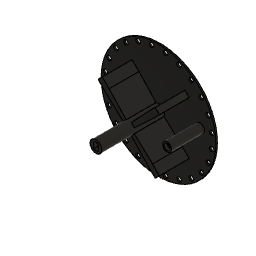
Assembly (Autodesk Fusion 360 archive; units mm, degrees)
design "Hour Wheel 2"
Autodesk Fusion 360 part; units mm, degrees
(part 1 of 2)
sketch "Sketch1" plane through (0, 0, 0) normal (0, 1, 0) x (1, 0, 0)
  circle A0 centre (0, 0) radius 38.5
  circle A1 centre (-4.6989, -35.692) radius 1.5
  circle A2 centre (4.6989, -35.692) radius 1.5
  circle A3 centre (13.7766, -33.2597) radius 1.5
  circle A4 centre (21.9154, -28.5607) radius 1.5
  circle A5 centre (28.5607, -21.9154) radius 1.5
  circle A6 centre (33.2597, -13.7766) radius 1.5
  circle A7 centre (35.692, -4.6989) radius 1.5
  circle A8 centre (35.692, 4.6989) radius 1.5
  circle A9 centre (33.2597, 13.7766) radius 1.5
  circle A10 centre (28.5607, 21.9154) radius 1.5
  circle A11 centre (21.9154, 28.5607) radius 1.5
  circle A12 centre (13.7766, 33.2597) radius 1.5
  circle A13 centre (4.6989, 35.692) radius 1.5
  circle A14 centre (-4.6989, 35.692) radius 1.5
  circle A15 centre (-13.7766, 33.2597) radius 1.5
  circle A16 centre (-21.9154, 28.5607) radius 1.5
  circle A17 centre (-28.5607, 21.9154) radius 1.5
  circle A18 centre (-33.2597, 13.7766) radius 1.5
  circle A19 centre (-35.692, 4.6989) radius 1.5
  circle A20 centre (-35.692, -4.6989) radius 1.5
  circle A21 centre (-33.2597, -13.7766) radius 1.5
  circle A22 centre (-28.5607, -21.9154) radius 1.5
  circle A23 centre (-21.9154, -28.5607) radius 1.5
  circle A24 centre (-13.7766, -33.2597) radius 1.5
  dimension "d1" = 77
  dimension "d2" = 3
  dimension "d3" = 36
  dimension "d5" = 360
  constraint coincident A0.centre origin
  measures "d1" diameter of A0
  measures "d2" diameter of A1
  measures "d3" distance of A0.centre A1.centre
extrude "Extrude1" add sketch "Sketch1" along normal blind 1 makes body 1
sketch "Sketch2" plane through (0, 0, 0) normal (0, 1, 0) x (1, 0, 0)
  line L0 (0, 0) -> (27.6586, 0) construction
  line L1 (0, 0) -> (41.0195, 0) construction
  line L2 (0, 0) -> (31, 0) construction
  line L3 (0, 0) -> (31, 0) construction
  line L4 (-15.9765, 13.148) -> (-13.148, 15.9765)
  line L5 (-14.5622, 14.5622) -> (-15.9765, 13.148)
  line L6 (-14.5622, 14.5622) -> (-13.148, 15.9765)
  line L7 (-15.9765, 13.148) -> (-20.5726, 17.7442)
  line L8 (-20.5726, 17.7442) -> (-17.7442, 20.5726)
  line L9 (-13.148, 15.9765) -> (-17.7442, 20.5726)
  line L10 (-15.9765, -13.148) -> (-20.5726, -17.7442)
  line L11 (-14.5622, -14.5622) -> (-13.148, -15.9765)
  line L12 (-13.148, -15.9765) -> (-17.7442, -20.5726)
  line L13 (-17.7442, -20.5726) -> (-20.5726, -17.7442)
  line L14 (-14.5622, -14.5622) -> (-15.9765, -13.148)
  line L15 (-13.148, -15.9765) -> (-15.9765, -13.148)
  line L16 (13.148, -15.9765) -> (17.7442, -20.5726)
  line L17 (14.5622, -14.5622) -> (15.9765, -13.148)
  line L18 (15.9765, -13.148) -> (20.5726, -17.7442)
  line L19 (20.5726, -17.7442) -> (17.7442, -20.5726)
  line L20 (14.5622, -14.5622) -> (13.148, -15.9765)
  line L21 (15.9765, -13.148) -> (13.148, -15.9765)
  line L22 (15.9765, 13.148) -> (20.5726, 17.7442)
  line L23 (14.5622, 14.5622) -> (13.148, 15.9765)
  line L24 (13.148, 15.9765) -> (17.7442, 20.5726)
  line L25 (17.7442, 20.5726) -> (20.5726, 17.7442)
  line L26 (14.5622, 14.5622) -> (15.9765, 13.148)
  line L27 (13.148, 15.9765) -> (15.9765, 13.148)
  line L28 (-15.9765, 13.148) -> (-3.6903, 1.691)
  line L29 (-15.9765, 13.148) -> (0.824, 13.148) construction
  line L30 (-13.148, 15.9765) -> (-1.7011, 3.7012)
  line L31 (-13.148, 15.9765) -> (3.6363, 15.9765) construction
  line L32 (13.148, 15.9765) -> (1.6437, 3.6396)
  line L33 (13.148, 15.9765) -> (30.0166, 15.9765) construction
  line L34 (15.9765, 13.148) -> (3.7292, 1.7273)
  line L35 (15.9765, 13.148) -> (32.7225, 13.148) construction
  line L36 (-15.9765, -13.148) -> (-3.6901, -1.6909)
  line L37 (-15.9765, -13.148) -> (0.8229, -13.148) construction
  line L38 (-13.148, -15.9765) -> (-1.6943, -3.6938)
  line L39 (-13.148, -15.9765) -> (3.6463, -15.9765) construction
  line L40 (15.9765, -13.148) -> (3.6446, -1.6484)
  line L41 (15.9765, -13.148) -> (32.8382, -13.148) construction
  line L42 (13.148, -15.9765) -> (1.6484, -3.6446)
  line L43 (13.148, -15.9765) -> (30.0097, -15.9765) construction
  arc A0 (3.6463, 1.6445) -> (1.6484, 3.6446) centre (0, 0) ccw
  arc A1 (1.6484, -3.6446) -> (3.6446, -1.6484) centre (0, 0) ccw
  arc A2 (-1.6458, 3.6457) -> (-3.6455, 1.6463) centre (0, 0) ccw
  arc A3 (-3.6455, -1.6463) -> (-1.6461, -3.6456) centre (0, 0) ccw
  line L44 (-3.6455, 1.6463) -> (-3.6903, 1.691)
  line L45 (-3.6901, -1.6909) -> (-3.6455, -1.6463)
  line L46 (1.9993, -0.0019) -> (1.9974, 0)
  line L47 (-1.6458, 3.6457) -> (-1.7011, 3.7012)
  line L48 (3.6463, 1.6445) -> (3.7292, 1.7273)
  line L49 (-1.6943, -3.6938) -> (-1.6461, -3.6456)
  line L50 (1.9993, -0.0019) -> (2.0012, 0)
  dimension "d26" = 2
  dimension "d27" = 2
  dimension "d28" = 6.5
  dimension "d29" = 4
  dimension "d30" = 27.0941
  dimension "d32" = 360
  dimension "d63" = 8
  dimension "d64" = 43
  dimension "d65" = 47
  dimension "d66" = 133
  dimension "d67" = 137
  dimension "d68" = 43
  dimension "d69" = 47
  dimension "d70" = 137
  dimension "d71" = 133
  constraint horizontal L0
  constraint coincident L0.start L1.start
  constraint horizontal L1
  constraint horizontal L2
  constraint horizontal L3
  constraint perpendicular L4 L7
  constraint perpendicular L8 L9
  constraint coincident L4 L5.start
  constraint horizontal L29
  constraint horizontal L31
  constraint horizontal L33
  constraint horizontal L35
  constraint horizontal L37
  constraint horizontal L39
  constraint horizontal L41
  constraint horizontal L43
  constraint coincident L42.end A2
  constraint coincident L32 A0.end
  constraint coincident A2.start L46
  constraint coincident A0.start L49
  constraint concentric A0 A2
  constraint concentric A1 A2
  constraint concentric A2 A3
  constraint collinear L46 L47
  constraint coincident L0 L50.end
  constraint collinear L48 L49
  constraint coincident L0 L46.end
  constraint coincident L46.start L49
  constraint collinear L49 L50
  measures "d26" distance of L5.start L4.start
  measures "d27" distance of L5.start L4.end
  measures "d28" distance of L4.start L7.end
  measures "d29" distance of L7.end L8.end
  measures "d30" distance of L0.start L8
  measures "d63" diameter of A2
  measures "d64" angle of L28 L29
  measures "d65" angle of L30 L31
  measures "d66" angle of L32 L33
  measures "d67" angle of L34 L35
  measures "d68" angle of L36 L37
  measures "d69" angle of L38 L39
  measures "d70" angle of L40 L41
  measures "d71" angle of L42 L43
extrude "Extrude2" add sketch "Sketch2" against normal blind 20 bodies 1
copy_body "Body->Comp1" bodies 1 removing the originals makes body 2 in component "Wheel"
sketch "Sketch3" plane through (0, 0, 0) normal (0, 1, 0) x (1, 0, 0)
  circle A0 centre (0, 0) radius 4
  dimension "d37" = 8
  constraint coincident A0.centre origin
  measures "d37" diameter of A0
extrude "Extrude1'" add sketch "Sketch3" against normal blind 42 bodies 2 in component "Wheel"
sketch "Sketch4" plane through (0, 0, 0) normal (0, 1, 0) x (1, 0, 0)
  line L0 (1.5, -2) -> (1.5, 2)
  line L1 (-1.5, 2) -> (-1.5, -2)
  arc A0 (-1.5, -2) -> (1.5, -2) centre (0, 0) ccw
  arc A1 (1.5, 2) -> (-1.5, 2) centre (0, 0) ccw
  dimension "d40" = 5
  dimension "d41" = 3
  dimension "d42" = 4
  constraint coincident A0.centre A1.centre
  constraint vertical L0
  constraint vertical L1
  constraint concentric A0 A1
  measures "d40" diameter of A0
  measures "d41" distance of L1.end L0.start
  measures "d42" distance of L1.end L1.start
extrude "Extrude2'" cut sketch "Sketch4" along normal blind 6.5 from surface at -42 bodies 2 in component "Wheel"
sketch "Sketch8" plane through (0, 0, 0) normal (0, 1, 0) x (1, 0, 0)
  line L0 (1.5, -1.5) -> (-1.5, -1.5)
  line L1 (-1.5, -1.5) -> (-1.5, 1.5)
  line L2 (-1.5, 1.5) -> (1.5, 1.5)
  line L3 (1.5, 1.5) -> (1.5, -1.5)
  dimension "d87" = 3
  dimension "d88" = 3
  dimension "d89" = 1.5
  dimension "d90" = 1.5
  constraint horizontal L0
  constraint vertical L1
  constraint horizontal L2
  constraint vertical L3
  measures "d87" distance of L0.start L0.end
  measures "d88" distance of L0.start L2.end
  measures "d89" distance of origin L3
  measures "d90" distance of origin L0
sketch "Sketch9" plane through (0, 0, 0) normal (0, 1, 0) x (1, 0, 0)
  circle A0 centre (0, 0) radius 10
  line L0 (0.6946, -3.9392) -> (1.5628, -8.8633)
  line L1 (4, 0) -> (9, 0) construction
  line L2 (3.9392, -0.6946) -> (8.8633, -1.5628)
  line L3 (4, 0) -> (9, 0) construction
  line L4 (-0.6946, -3.9392) -> (-1.5628, -8.8633)
  line L5 (4, 0) -> (9, 0) construction
  line L6 (-3.9392, -0.6946) -> (-8.8633, -1.5628)
  line L7 (4, 0) -> (9, 0) construction
  line L8 (-3.9392, 0.6946) -> (-8.8633, 1.5628)
  line L9 (4, 0) -> (9, 0) construction
  line L10 (3.9392, 0.6946) -> (8.8633, 1.5628)
  line L11 (4, 0) -> (9, 0) construction
  line L12 (-0.6946, 3.9392) -> (-1.5628, 8.8633)
  line L13 (0.6946, 3.9392) -> (1.5628, 8.8633)
  arc A1 (8.8633, 1.5628) -> (1.5628, 8.8633) centre (0, 0) ccw
  arc A2 (-1.5628, 8.8633) -> (-8.8633, 1.5628) centre (0, 0) ccw
  arc A3 (-8.8633, -1.5628) -> (-1.5628, -8.8633) centre (0, 0) ccw
  arc A4 (1.5628, -8.8633) -> (8.8633, -1.5628) centre (0, 0) ccw
  arc A5 (3.9392, 0.6946) -> (0.6946, 3.9392) centre (0, 0) ccw
  arc A6 (-0.6946, 3.9392) -> (-3.9392, 0.6946) centre (0, 0) ccw
  arc A7 (-3.9392, -0.6946) -> (-0.6946, -3.9392) centre (0, 0) ccw
  arc A8 (0.6946, -3.9392) -> (3.9392, -0.6946) centre (0, 0) ccw
  dimension "d81" = 80
  dimension "d82" = 10
  dimension "d83" = 100
  dimension "d84" = 170
  dimension "d85" = 170
  dimension "d86" = 10
  constraint horizontal L1
  constraint horizontal L3
  constraint horizontal L5
  constraint horizontal L7
  constraint horizontal L9
  constraint horizontal L11
  constraint coincident L12.end A1
  constraint parallel L0 L12
  constraint perpendicular L8 L13
  constraint concentric A1 A2
  constraint concentric A2 A3
  constraint concentric A3 A4
  constraint concentric A1 A5
  constraint coincident L4.start A5
  constraint coincident L6.start A5
  constraint coincident L8.start A5
  constraint coincident L12.start A5
  constraint concentric A5 A6
  constraint concentric A6 A7
  constraint coincident A0.centre A1.centre
  measures "d81" angle of L0 L1
  measures "d82" angle of L2 L3
  measures "d83" angle of L4 L5
  measures "d84" angle of L6 L7
  measures "d85" angle of L8 L9
  measures "d86" angle of L10 L11
extrude "Extrude5" cut sketch "Sketch8" against normal blind 10 from surface at 2 bodies 2 in component "Wheel"
sketch "Sketch10" plane through (0, 0, 0) normal (0, -1, 0) x (1, 0, 0)
  arc A0 (-1.6458, -3.6457) -> (1.6484, -3.6446) centre (0, 0) ccw
  line L0 (-1.6458, -3.6457) -> (-1.7011, -3.7012)
  line L1 (-1.7011, -3.7012) -> (-13.148, -15.9765)
  line L2 (-13.148, -15.9765) -> (-17.7442, -20.5726)
  line L3 (-17.7442, -20.5726) -> (-20.5726, -17.7442)
  line L4 (-20.5726, -17.7442) -> (-15.9765, -13.148)
  line L5 (-15.9765, -13.148) -> (-3.6903, -1.691)
  line L6 (-3.6903, -1.691) -> (-3.6455, -1.6463)
  arc A1 (-3.6455, 1.6463) -> (-3.6455, -1.6463) centre (0, 0) ccw
  line L7 (-3.6455, 1.6463) -> (-3.6901, 1.6909)
  line L8 (-3.6901, 1.6909) -> (-15.9765, 13.148)
  line L9 (-15.9765, 13.148) -> (-20.5726, 17.7442)
  line L10 (-20.5726, 17.7442) -> (-17.7442, 20.5726)
  line L11 (-17.7442, 20.5726) -> (-13.148, 15.9765)
  line L12 (-13.148, 15.9765) -> (-1.6943, 3.6938)
  line L13 (-1.6943, 3.6938) -> (-1.6461, 3.6456)
  arc A2 (1.6484, 3.6446) -> (-1.6461, 3.6456) centre (0, 0) ccw
  line L14 (1.6484, 3.6446) -> (13.148, 15.9765)
  line L15 (13.148, 15.9765) -> (17.7442, 20.5726)
  line L16 (17.7442, 20.5726) -> (20.5726, 17.7442)
  line L17 (20.5726, 17.7442) -> (15.9765, 13.148)
  line L18 (15.9765, 13.148) -> (3.6446, 1.6484)
  arc A3 (3.6463, -1.6445) -> (3.6446, 1.6484) centre (0, 0) ccw
  line L19 (3.6463, -1.6445) -> (3.7292, -1.7273)
  line L20 (3.7292, -1.7273) -> (15.9765, -13.148)
  line L21 (15.9765, -13.148) -> (20.5726, -17.7442)
  line L22 (20.5726, -17.7442) -> (17.7442, -20.5726)
  line L23 (17.7442, -20.5726) -> (13.148, -15.9765)
  line L24 (13.148, -15.9765) -> (1.6484, -3.6446)
  circle A4 centre (-35.692, -4.6989) radius 1.5
  circle A5 centre (-33.2597, 13.7766) radius 1.5
  circle A6 centre (-28.5607, 21.9154) radius 1.5
  circle A7 centre (-21.9154, 28.5607) radius 1.5
  circle A8 centre (-13.7766, 33.2597) radius 1.5
  circle A9 centre (-35.692, 4.6989) radius 1.5
  circle A10 centre (-33.2597, -13.7766) radius 1.5
  circle A11 centre (-28.5607, -21.9154) radius 1.5
  circle A12 centre (-21.9154, -28.5607) radius 1.5
  circle A13 centre (-13.7766, -33.2597) radius 1.5
  circle A14 centre (4.6989, -35.692) radius 1.5
  circle A15 centre (-4.6989, -35.692) radius 1.5
  circle A16 centre (13.7766, -33.2597) radius 1.5
  circle A17 centre (21.9154, -28.5607) radius 1.5
  circle A18 centre (28.5607, -21.9154) radius 1.5
  circle A19 centre (33.2597, -13.7766) radius 1.5
  circle A20 centre (35.692, -4.6989) radius 1.5
  circle A21 centre (35.692, 4.6989) radius 1.5
  circle A22 centre (33.2597, 13.7766) radius 1.5
  circle A23 centre (28.5607, 21.9154) radius 1.5
  circle A24 centre (21.9154, 28.5607) radius 1.5
  circle A25 centre (13.7766, 33.2597) radius 1.5
  circle A26 centre (4.6989, 35.692) radius 1.5
  circle A27 centre (-4.6989, 35.692) radius 1.5
  circle A28 centre (0, 0) radius 38.5
  circle A29 centre (27.7605, 3.6547) radius 3
  dimension "d91" = 8
  dimension "d92" = 6
  measures "d91" distance of A21.centre A29.centre
  measures "d92" diameter of A29
extrude "Extrude7" add sketch "Sketch10" along normal blind 22 contours A29 bodies 2 in component "Wheel"
sketch "Sketch11" plane through (0, -22, 0) normal (0, -1, 0) x (1, 0, 0)
  circle A0 centre (27.7605, 3.6547) radius 3
  circle A1 centre (27.7605, 3.6547) radius 2
  dimension "d96" = 4
  constraint concentric A0 A1
  measures "d96" diameter of A1
extrude "Extrude8" cut sketch "Sketch11" against normal blind 2 contours A1 bodies 2 in component "Wheel"
component "Wheel" placed x (1, 0, 0) y (0, 1, 0) z (0, 0, 1) at (0, 0, 0)

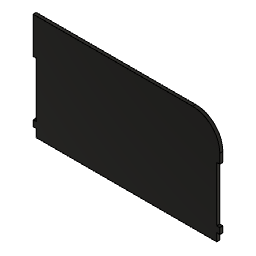
design "Minute Flap"
Autodesk Fusion 360 part; units mm, degrees
sketch "Sketch1" plane through (0, 0, 0) normal (0, 1, 0) x (1, 0, 0)
  line L0 (1, 0) -> (61, 0)
  line L1 (53, -35) -> (0, -35)
  arc A0 (53, -35) -> (62, -26) centre (53, -26) ccw
  line L2 (0, -2.6) -> (1, -2.6)
  line L3 (1, -4.6) -> (0, -4.6)
  line L4 (0, -4.6) -> (0, -2.6)
  line L5 (1, -2.6) -> (1, 0)
  line L6 (1, -4.6) -> (1, -22.85)
  line L7 (1, -22.85) -> (0, -22.85)
  line L8 (0, -35) -> (0, -22.85)
  line L9 (0, -4.6) -> (0, -2.6)
  line L10 (61, -22.85) -> (62, -22.85)
  line L11 (61, -4.6) -> (62, -4.6)
  line L12 (61, -2.6) -> (62, -2.6)
  line L13 (61, -2.6) -> (61, 0)
  line L14 (61, -4.6) -> (61, -22.85)
  line L15 (62, -2.6) -> (62, -4.6)
  line L16 (62, -22.85) -> (62, -26)
  dimension "d2" = 35
  dimension "d3" = 9
  dimension "d4" = 1
  dimension "d5" = 2
  dimension "d6" = 2.6
  dimension "d7" = 18.25
  dimension "d9" = 2.6
  dimension "d10" = 2
  dimension "d11" = 18.25
  dimension "d14" = 53
  dimension "d15" = 1
  dimension "d16" = 1
  constraint horizontal L0
  constraint vertical L15
  constraint horizontal L1
  constraint vertical L8
  constraint tangent L1 A0
  constraint tangent A0 L15
  constraint horizontal L2
  constraint horizontal L3
  constraint vertical L4
  constraint perpendicular L0 L5
  constraint perpendicular L3 L6
  constraint perpendicular L7 L8
  constraint collinear L8 L9
  constraint coincident L10.end L15
  constraint perpendicular L10 L15
  constraint perpendicular L11 L15
  constraint perpendicular L12 L15
  constraint perpendicular L0 L13
  constraint perpendicular L10 L14
  constraint collinear L15 L16
  measures "d2" distance of origin L1.end
  measures "d3" radius of A0
  measures "d4" distance of L2.start L2.end
  measures "d5" distance of L2.start L3.end
  measures "d6" distance of L0 L2
  measures "d7" distance of L3.start L6.end
  measures "d9" distance of L12.start L0.end
  measures "d10" distance of L12.start L11.start
  measures "d11" distance of L11.start L10.start
  measures "d14" distance of L1.end L1.start
  measures "d15" distance of L10.end L10.start
  measures "d16" distance of L12.end L12.start
extrude "Extrude1" add sketch "Sketch1" along normal blind 1 makes body 1
copy_body "Body->Comp1" bodies 1 removing the originals makes body 2 in component "Flap"
component "Flap" placed x (1, 0, 0) y (0, 1, 0) z (0, 0, 1) at (0, 0, 0)

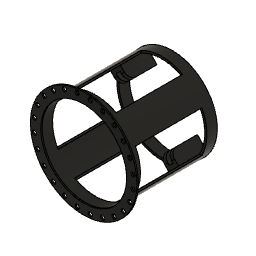
design "Hour Wheel 1"
Autodesk Fusion 360 part; units mm, degrees
sketch "Sketch1" plane through (0, 0, 0) normal (0, 1, 0) x (1, 0, 0)
  circle A0 centre (49.9693, -49.8433) radius 38.5
  circle A1 centre (45.2704, -85.5353) radius 1.5
  circle A2 centre (54.6683, -85.5353) radius 1.5
  circle A3 centre (63.7459, -83.103) radius 1.5
  circle A4 centre (71.8847, -78.404) radius 1.5
  circle A5 centre (78.53, -71.7587) radius 1.5
  circle A6 centre (83.229, -63.6199) radius 1.5
  circle A7 centre (85.6613, -54.5423) radius 1.5
  circle A8 centre (85.6613, -45.1444) radius 1.5
  circle A9 centre (83.229, -36.0667) radius 1.5
  circle A10 centre (78.53, -27.9279) radius 1.5
  circle A11 centre (71.8847, -21.2826) radius 1.5
  circle A12 centre (63.7459, -16.5837) radius 1.5
  circle A13 centre (54.6683, -14.1513) radius 1.5
  circle A14 centre (45.2704, -14.1513) radius 1.5
  circle A15 centre (36.1927, -16.5837) radius 1.5
  circle A16 centre (28.0539, -21.2826) radius 1.5
  circle A17 centre (21.4086, -27.9279) radius 1.5
  circle A18 centre (16.7096, -36.0667) radius 1.5
  circle A19 centre (14.2773, -45.1444) radius 1.5
  circle A20 centre (14.2773, -54.5423) radius 1.5
  circle A21 centre (16.7096, -63.6199) radius 1.5
  circle A22 centre (21.4086, -71.7587) radius 1.5
  circle A23 centre (28.0539, -78.404) radius 1.5
  circle A24 centre (36.1927, -83.103) radius 1.5
  circle A25 centre (49.9693, -49.8433) radius 31
  dimension "d1" = 77
  dimension "d2" = 3
  dimension "d3" = 36
  dimension "d5" = 360
  dimension "d6" = 62
  constraint concentric A0 A25
  measures "d1" diameter of A0
  measures "d2" diameter of A1
  measures "d3" distance of A0.centre A1.centre
  measures "d6" diameter of A25
extrude "Extrude1" add sketch "Sketch1" along normal blind 1 makes body 1
sketch "Sketch2" plane through (0, 0, 0) normal (0, -1, 0) x (1, 0, 0)
  circle A0 centre (16.7096, 63.6199) radius 1.5
  circle A1 centre (21.4086, 71.7587) radius 1.5
  circle A2 centre (28.0539, 78.404) radius 1.5
  circle A3 centre (36.1927, 83.103) radius 1.5
  circle A4 centre (49.9693, 49.8433) radius 31
  circle A5 centre (54.6683, 14.1513) radius 1.5
  circle A6 centre (45.2704, 14.1513) radius 1.5
  circle A7 centre (36.1927, 16.5837) radius 1.5
  circle A8 centre (28.0539, 21.2826) radius 1.5
  circle A9 centre (21.4086, 27.9279) radius 1.5
  circle A10 centre (16.7096, 36.0667) radius 1.5
  circle A11 centre (14.2773, 45.1444) radius 1.5
  circle A12 centre (14.2773, 54.5423) radius 1.5
  circle A13 centre (63.7459, 16.5837) radius 1.5
  circle A14 centre (71.8847, 21.2826) radius 1.5
  circle A15 centre (78.53, 27.9279) radius 1.5
  circle A16 centre (83.229, 36.0667) radius 1.5
  circle A17 centre (85.6613, 45.1444) radius 1.5
  circle A18 centre (85.6613, 54.5423) radius 1.5
  circle A19 centre (83.229, 63.6199) radius 1.5
  circle A20 centre (78.53, 71.7587) radius 1.5
  circle A21 centre (71.8847, 78.404) radius 1.5
  circle A22 centre (63.7459, 83.103) radius 1.5
  circle A23 centre (54.6683, 85.5353) radius 1.5
  circle A24 centre (45.2704, 85.5353) radius 1.5
  circle A25 centre (49.9693, 49.8433) radius 38.5
sketch "Sketch3" plane through (0, 0, 0) normal (0, -1, 0) x (1, 0, 0)
  circle A0 centre (50, 50) radius 32.5
  circle A1 centre (50, 50) radius 31
  dimension "d10" = 65
  dimension "d22" = 62
  constraint concentric A0 A1
  measures "d10" diameter of A0
  measures "d22" diameter of A1
extrude "Extrude4" add sketch "Sketch3" against normal blind 63 from surface at -1 separate body makes body 2
sketch "Sketch5" plane through (0, 0, 0) normal (1, 0, 0) x (0, 1, 0)
  line L0 (8.5, 64.8433) -> (56.5, 64.8433)
  line L1 (56.5, 64.8433) -> (56.5, 34.8433)
  line L2 (56.5, 34.8433) -> (8.5, 34.8433)
  line L3 (8.5, 34.8433) -> (8.5, 64.8433)
  line L4 (1, 11.5) -> (1, 50)
  line L5 (1, 11.3433) -> (1, 88.3433)
  point P0 (1, 49.8433)
  dimension "d23" = 48
  dimension "d24" = 30
  dimension "d25" = 38.5
  dimension "d26" = 15
  dimension "d29" = 7.5
  constraint horizontal L0
  constraint vertical L1
  constraint horizontal L2
  constraint vertical L3
  constraint vertical L4
  measures "d23" distance of L0.start L0.end
  measures "d24" distance of L0.end L1.end
  measures "d25" distance of L4.start L4.end
  measures "d26" vertical distance of L2.end P0
  measures "d29" distance of L3 L5
extrude "Extrude5" cut sketch "Sketch5" along normal blind 100 bodies 2
sketch "Sketch6" plane through (0, 0, 0) normal (0, 0, 1) x (1, 0, 0)
  line L0 (34.9693, 56.5) -> (64.9693, 56.5)
  line L1 (64.9693, 56.5) -> (64.9693, 8.5)
  line L2 (64.9693, 8.5) -> (34.9693, 8.5)
  line L3 (34.9693, 8.5) -> (34.9693, 56.5)
  line L4 (88.4693, 1) -> (11.4693, 1)
  line L5 (88.4693, 1) -> (49.9693, 1)
  dimension "d30" = 30
  dimension "d31" = 48
  dimension "d32" = 7.5
  dimension "d33" = 38.5
  dimension "d34" = 15
  constraint horizontal L0
  constraint vertical L1
  constraint horizontal L2
  constraint vertical L3
  constraint coincident L4.start L5.start
  constraint parallel L4 L5
  measures "d30" distance of L0.start L0.end
  measures "d31" distance of L0.end L1.end
  measures "d32" distance of L2 L4
  measures "d33" distance of L4.start L5.end
  measures "d34" horizontal distance of L1.end L5.end
extrude "Extrude6" cut sketch "Sketch6" along normal blind 95 bodies 2
copy_body "Body->Comp5" bodies 1 removing the originals makes body 3 in component "Wheel"
copy_body "Body->Comp6" bodies 2 removing the originals makes body 4 in component "Axis"
sketch "Sketch11" plane through (0, 64, 0) normal (0, 1, 0) x (-1, 0, 0)
  circle A0 centre (0.0307, -0.1567) radius 31
  circle A1 centre (0.0307, -0.1567) radius 32.5
  line L0 (0.0307, -0.1567) -> (31.0307, -0.1567) construction
  line L1 (18.1285, -25.3255) -> (11.0574, -18.2544)
  line L2 (25.1995, -18.2544) -> (18.1285, -11.1834)
  arc A2 (18.1285, -25.3255) -> (25.1995, -18.2544) centre (0.0307, -0.1567) ccw
  line L3 (25.1995, -18.2544) -> (18.1285, -11.1834)
  line L4 (13.1787, -16.1331) -> (17.7749, -20.7293)
  line L5 (17.7749, -20.7293) -> (20.6033, -17.9009)
  line L6 (20.6033, -17.9009) -> (16.0071, -13.3047)
  line L7 (18.1285, -11.1834) -> (16.0071, -13.3047)
  line L8 (13.1787, -16.1331) -> (11.0574, -18.2544)
  line L9 (18.1285, 25.0122) -> (11.0574, 17.9411)
  line L10 (16.0071, 12.9914) -> (18.1285, 10.87)
  line L11 (17.7749, 20.416) -> (13.1787, 15.8198)
  arc A3 (25.1995, 17.9411) -> (18.1285, 25.0122) centre (0.0307, -0.1567) ccw
  line L12 (20.6033, 17.5875) -> (17.7749, 20.416)
  line L13 (11.0574, 17.9411) -> (13.1787, 15.8198)
  line L14 (25.1995, 17.9411) -> (18.1285, 10.87)
  line L15 (16.0071, 12.9914) -> (20.6033, 17.5875)
  line L16 (18.1285, 25.0122) -> (11.0574, 17.9411)
  line L17 (-25.1381, 17.9411) -> (-18.0671, 10.87)
  line L18 (-13.1173, 15.8198) -> (-10.996, 17.9411)
  line L19 (-20.542, 17.5875) -> (-15.9458, 12.9914)
  arc A4 (-18.0671, 25.0122) -> (-25.1381, 17.9411) centre (0.0307, -0.1567) ccw
  line L20 (-17.7135, 20.416) -> (-20.542, 17.5875)
  line L21 (-18.0671, 10.87) -> (-15.9458, 12.9914)
  line L22 (-18.0671, 25.0122) -> (-10.996, 17.9411)
  line L23 (-13.1173, 15.8198) -> (-17.7135, 20.416)
  line L24 (-25.1381, 17.9411) -> (-18.0671, 10.87)
  line L25 (-18.0671, -25.3255) -> (-10.996, -18.2544)
  line L26 (-15.9458, -13.3047) -> (-18.0671, -11.1834)
  line L27 (-17.7135, -20.7293) -> (-13.1173, -16.1331)
  arc A5 (-25.1381, -18.2544) -> (-18.0671, -25.3255) centre (0.0307, -0.1567) ccw
  line L28 (-20.542, -17.9009) -> (-17.7135, -20.7293)
  line L29 (-10.996, -18.2544) -> (-13.1173, -16.1331)
  line L30 (-25.1381, -18.2544) -> (-18.0671, -11.1834)
  line L31 (-15.9458, -13.3047) -> (-20.542, -17.9009)
  line L32 (-18.0671, -25.3255) -> (-10.996, -18.2544)
  dimension "d107" = 10
  dimension "d108" = 6.5
  dimension "d109" = 4
  dimension "d110" = 3
  dimension "d111" = 3
  dimension "d112" = 6.5
  dimension "d114" = 360
  constraint concentric A0 A2
  constraint horizontal L0
  constraint coincident A0.centre A1.centre
  constraint coincident A0 L2.start
  constraint coincident A0 L1.start
  constraint parallel L2 L3
  constraint perpendicular L1 L7
  constraint coincident L4.start L7
  constraint perpendicular L4 L7
  constraint perpendicular L6 L7
  constraint collinear L7 L8
  measures "d107" distance of L2.start L2.end
  measures "d108" distance of L4.start L4.end
  measures "d109" distance of L4.end L5.end
  measures "d110" distance of L1 L4
  measures "d111" distance of L2 L6
  measures "d112" distance of L5.end L6.end
extrude "Extrude1'" add sketch "Sketch11" against normal blind 20 contours A0 L9 L10 L11 A3 L12 L13 L14 L15 L16 | A0 L1 L2 A2 L3 L4 L5 L6 L7 L8 | A0 L17 L18 L19 A4 L20 L21 L22 L23 L24 | A0 L25 L26 L27 A5 L28 L29 L30 L31 L32 sketch seen with x (1, 0, 0) y (0, 1, 0) z (0, 0, 1) at (50.0307, 0, 50.1567) bodies 4 in component "Axis"
fillet "Fillet1" radius 5 8 edges at (37.9126, 44, 67.0371) (32.9629, 44, 62.0874) (32.9629, 44, 37.9126) (37.9126, 44, 32.9629) (67.0371, 44, 37.9126) (62.0874, 44, 32.9629) (62.0874, 44, 67.0371) (67.0371, 44, 62.0874) on bodies 4 in component "Axis"
component "Wheel" placed x (1, 0, 0) y (0, 1, 0) z (0, 0, 1) at (-50, 0, -50)
component "Axis" placed x (1, 0, 0) y (0, 1, 0) z (0, 0, 1) at (-50.0307, 0, -50.1567)
equation "d25 = ( 77 / 2 ) * 1 mm"
equation "d33 = ( 77 / 2 ) * 1 mm"

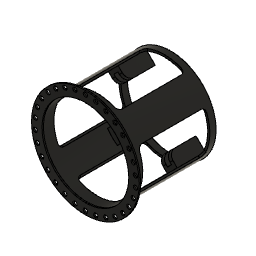
design "Minute Wheel 1"
Autodesk Fusion 360 part; units mm, degrees
sketch "Sketch1" plane through (0, 0, 0) normal (0, 1, 0) x (1, 0, 0)
  circle A0 centre (50, -49.5) radius 38.5
  circle A1 centre (50, -49.5) radius 31
  circle A2 centre (50, -85.5) radius 1.5
  circle A3 centre (57.4848, -84.7133) radius 1.5
  circle A4 centre (64.6425, -82.3876) radius 1.5
  circle A5 centre (71.1603, -78.6246) radius 1.5
  circle A6 centre (76.7532, -73.5887) radius 1.5
  circle A7 centre (81.1769, -67.5) radius 1.5
  circle A8 centre (84.238, -60.6246) radius 1.5
  circle A9 centre (85.8028, -53.263) radius 1.5
  circle A10 centre (85.8028, -45.737) radius 1.5
  circle A11 centre (84.238, -38.3754) radius 1.5
  circle A12 centre (81.1769, -31.5) radius 1.5
  circle A13 centre (76.7532, -25.4113) radius 1.5
  circle A14 centre (71.1603, -20.3754) radius 1.5
  circle A15 centre (64.6425, -16.6124) radius 1.5
  circle A16 centre (57.4848, -14.2867) radius 1.5
  circle A17 centre (50, -13.5) radius 1.5
  circle A18 centre (42.5152, -14.2867) radius 1.5
  circle A19 centre (35.3575, -16.6124) radius 1.5
  circle A20 centre (28.8397, -20.3754) radius 1.5
  circle A21 centre (23.2468, -25.4113) radius 1.5
  circle A22 centre (18.8231, -31.5) radius 1.5
  circle A23 centre (15.762, -38.3754) radius 1.5
  circle A24 centre (14.1972, -45.737) radius 1.5
  circle A25 centre (14.1972, -53.263) radius 1.5
  circle A26 centre (15.762, -60.6246) radius 1.5
  circle A27 centre (18.8231, -67.5) radius 1.5
  circle A28 centre (23.2468, -73.5887) radius 1.5
  circle A29 centre (28.8397, -78.6246) radius 1.5
  circle A30 centre (35.3575, -82.3876) radius 1.5
  circle A31 centre (42.5152, -84.7133) radius 1.5
  dimension "d1" = 77
  dimension "d6" = 62
  dimension "d86" = 3
  dimension "d87" = 36
  dimension "d89" = 360
  constraint concentric A0 A1
  measures "d1" diameter of A0
  measures "d6" diameter of A1
  measures "d86" diameter of A2
  measures "d87" distance of A0.centre A2.centre
extrude "Extrude1" add sketch "Sketch1" along normal blind 1 makes body 1
sketch "Sketch2" plane through (0, 0, 0) normal (0, -1, 0) x (1, 0, 0)
  circle A0 centre (50, 49.5) radius 31
  circle A1 centre (50, 49.5) radius 38.5
  circle A2 centre (18.8231, 67.5) radius 1.5
  circle A3 centre (35.3575, 82.3876) radius 1.5
  circle A4 centre (64.6425, 16.6124) radius 1.5
  circle A5 centre (23.2468, 73.5887) radius 1.5
  circle A6 centre (28.8397, 78.6246) radius 1.5
  circle A7 centre (14.1972, 53.263) radius 1.5
  circle A8 centre (15.762, 60.6246) radius 1.5
  circle A9 centre (42.5152, 14.2867) radius 1.5
  circle A10 centre (50, 13.5) radius 1.5
  circle A11 centre (57.4848, 14.2867) radius 1.5
  circle A12 centre (42.5152, 84.7133) radius 1.5
  circle A13 centre (35.3575, 16.6124) radius 1.5
  circle A14 centre (28.8397, 20.3754) radius 1.5
  circle A15 centre (23.2468, 25.4113) radius 1.5
  circle A16 centre (18.8231, 31.5) radius 1.5
  circle A17 centre (15.762, 38.3754) radius 1.5
  circle A18 centre (14.1972, 45.737) radius 1.5
  circle A19 centre (71.1603, 20.3754) radius 1.5
  circle A20 centre (76.7532, 25.4113) radius 1.5
  circle A21 centre (81.1769, 31.5) radius 1.5
  circle A22 centre (84.238, 38.3754) radius 1.5
  circle A23 centre (85.8028, 45.737) radius 1.5
  circle A24 centre (85.8028, 53.263) radius 1.5
  circle A25 centre (84.238, 60.6246) radius 1.5
  circle A26 centre (81.1769, 67.5) radius 1.5
  circle A27 centre (76.7532, 73.5887) radius 1.5
  circle A28 centre (71.1603, 78.6246) radius 1.5
  circle A29 centre (64.6425, 82.3876) radius 1.5
  circle A30 centre (57.4848, 84.7133) radius 1.5
  circle A31 centre (50, 85.5) radius 1.5
sketch "Sketch3" plane through (0, 0, 0) normal (0, -1, 0) x (1, 0, 0)
  circle A0 centre (50, 50) radius 32.5
  circle A1 centre (50, 50) radius 31
  dimension "d10" = 65
  dimension "d22" = 62
  constraint concentric A0 A1
  measures "d10" diameter of A0
  measures "d22" diameter of A1
extrude "Extrude4" add sketch "Sketch3" against normal blind 60 from surface at -1 separate body makes body 2
sketch "Sketch5" plane through (0, 0, 0) normal (1, 0, 0) x (0, 1, 0)
  line L0 (11.5, 64.5) -> (53.5, 64.5)
  line L1 (56.5, 61.5) -> (56.5, 37.5)
  line L2 (53.5, 34.5) -> (11.5, 34.5)
  line L3 (8.5, 37.5) -> (8.5, 61.5)
  line L4 (1, 11.5) -> (1, 50)
  line L5 (1, 11) -> (1, 88)
  arc A0 (56.5, 61.5) -> (53.5, 64.5) centre (53.5, 61.5) ccw
  arc A1 (11.5, 64.5) -> (8.5, 61.5) centre (11.5, 61.5) ccw
  arc A2 (53.5, 34.5) -> (56.5, 37.5) centre (53.5, 37.5) ccw
  arc A3 (8.5, 37.5) -> (11.5, 34.5) centre (11.5, 37.5) ccw
  point P0 (8.5, 64.5)
  point P1 (56.5, 64.5)
  point P2 (56.5, 34.5)
  point P3 (8.5, 34.5)
  point P4 (1, 49.5)
  dimension "d23" = 48
  dimension "d24" = 30
  dimension "d25" = 38.5
  dimension "d26" = 15
  dimension "d29" = 7.5
  dimension "d94" = 3
  dimension "d95" = 3
  dimension "d96" = 3
  dimension "d97" = 3
  constraint horizontal L0
  constraint vertical L1
  constraint horizontal L2
  constraint vertical L3
  constraint vertical L4
  constraint coincident P1 L0
  constraint coincident P1 L1
  constraint tangent L0 A0
  constraint tangent L1 A0
  constraint coincident P0 L0
  constraint coincident P0 L3
  constraint tangent L0 A1
  constraint tangent L3 A1
  constraint coincident P2 L1
  constraint coincident P2 L2
  constraint tangent L1 A2
  constraint tangent L2 A2
  constraint coincident P3 L3
  constraint coincident P3 L2
  constraint tangent L3 A3
  constraint tangent L2 A3
  measures "d23" distance of P0 P1
  measures "d24" distance of P1 P2
  measures "d25" distance of L4.start L4.end
  measures "d26" vertical distance of P3 P4
  measures "d29" distance of L3 L5
  measures "d94" radius of A0
  measures "d95" radius of A1
  measures "d96" radius of A2
  measures "d97" radius of A3
extrude "Extrude5" cut sketch "Sketch5" along normal blind 100 bodies 2
sketch "Sketch6" plane through (0, 0, 0) normal (0, 0, 1) x (1, 0, 0)
  line L0 (38, 56.5) -> (62, 56.5)
  line L1 (65, 53.5) -> (65, 11.5)
  line L2 (62, 8.5) -> (38, 8.5)
  line L3 (35, 11.5) -> (35, 53.5)
  line L4 (88.5, 1) -> (11.5, 1)
  line L5 (88.5, 1) -> (50, 1)
  arc A0 (35, 11.5) -> (38, 8.5) centre (38, 11.5) ccw
  arc A1 (62, 8.5) -> (65, 11.5) centre (62, 11.5) ccw
  arc A2 (38, 56.5) -> (35, 53.5) centre (38, 53.5) ccw
  arc A3 (65, 53.5) -> (62, 56.5) centre (62, 53.5) ccw
  point P0 (35, 56.5)
  point P1 (65, 56.5)
  point P2 (65, 8.5)
  dimension "d30" = 30
  dimension "d31" = 48
  dimension "d32" = 7.5
  dimension "d33" = 38.5
  dimension "d34" = 15
  dimension "d90" = 3
  dimension "d91" = 3
  dimension "d92" = 3
  dimension "d93" = 3
  constraint horizontal L0
  constraint vertical L1
  constraint horizontal L2
  constraint vertical L3
  constraint coincident L4.start L5.start
  constraint parallel L4 L5
  constraint tangent L3 A0
  constraint tangent L2 A0
  constraint coincident P2 L1
  constraint coincident P2 L2
  constraint tangent L1 A1
  constraint tangent L2 A1
  constraint coincident P0 L0
  constraint coincident P0 L3
  constraint tangent L0 A2
  constraint tangent L3 A2
  constraint coincident P1 L0
  constraint coincident P1 L1
  constraint tangent L0 A3
  constraint tangent L1 A3
  measures "d30" distance of P0 P1
  measures "d31" distance of P1 P2
  measures "d32" distance of L2 L4
  measures "d33" distance of L4.start L5.end
  measures "d34" horizontal distance of P2 L5.end
  measures "d90" radius of A0
  measures "d91" radius of A1
  measures "d92" radius of A2
  measures "d93" radius of A3
extrude "Extrude6" cut sketch "Sketch6" along normal blind 95 bodies 2
copy_body "Body->Comp5" bodies 2 removing the originals makes body 3 in component "Axis"
copy_body "Body->Comp6" bodies 1 removing the originals makes body 4 in component "Wheel"
sketch "Sketch9" plane through (0, 0, 0) normal (0, 1, 0) x (1, 0, 0)
  line L0 (50, -50) -> (81, -50) construction
  line L1 (31.9022, -24.8312) -> (38.9733, -31.9022)
  line L2 (24.8312, -31.9022) -> (31.9022, -38.9733)
  line L3 (36.852, -34.0235) -> (32.2558, -29.4274)
  line L4 (32.2558, -29.4274) -> (29.4274, -32.2558)
  line L5 (29.4274, -32.2558) -> (34.0235, -36.852)
  line L6 (31.9022, -38.9733) -> (34.0235, -36.852)
  line L7 (36.852, -34.0235) -> (38.9733, -31.9022)
  arc A0 (31.9022, -24.8312) -> (24.8312, -31.9022) centre (50, -50) ccw
  line L8 (31.9022, -75.1688) -> (38.9733, -68.0978)
  line L9 (32.2558, -70.5726) -> (36.852, -65.9765)
  line L10 (29.4274, -67.7442) -> (32.2558, -70.5726)
  line L11 (34.0235, -63.148) -> (29.4274, -67.7442)
  line L12 (24.8312, -68.0978) -> (31.9022, -61.0267)
  line L13 (34.0235, -63.148) -> (31.9022, -61.0267)
  line L14 (38.9733, -68.0978) -> (36.852, -65.9765)
  arc A1 (24.8312, -68.0978) -> (31.9022, -75.1688) centre (50, -50) ccw
  line L15 (75.1688, -68.0978) -> (68.0978, -61.0267)
  line L16 (70.5726, -67.7442) -> (65.9765, -63.148)
  line L17 (67.7442, -70.5726) -> (70.5726, -67.7442)
  line L18 (63.148, -65.9765) -> (67.7442, -70.5726)
  line L19 (68.0978, -75.1688) -> (61.0267, -68.0978)
  line L20 (63.148, -65.9765) -> (61.0267, -68.0978)
  line L21 (68.0978, -61.0267) -> (65.9765, -63.148)
  arc A2 (68.0978, -75.1688) -> (75.1688, -68.0978) centre (50, -50) ccw
  line L22 (68.0978, -24.8312) -> (61.0267, -31.9022)
  line L23 (67.7442, -29.4274) -> (63.148, -34.0235)
  line L24 (70.5726, -32.2558) -> (67.7442, -29.4274)
  line L25 (65.9765, -36.852) -> (70.5726, -32.2558)
  line L26 (75.1688, -31.9022) -> (68.0978, -38.9733)
  line L27 (65.9765, -36.852) -> (68.0978, -38.9733)
  line L28 (61.0267, -31.9022) -> (63.148, -34.0235)
  arc A3 (75.1688, -31.9022) -> (68.0978, -24.8312) centre (50, -50) ccw
  dimension "d138" = 62
  dimension "d147" = 10
  dimension "d148" = 6.5
  dimension "d149" = 4
  dimension "d150" = 3
  dimension "d151" = 3
  dimension "d152" = 4
  dimension "d153" = 6.5
  dimension "d154" = 10
  dimension "d156" = 360
  constraint horizontal L0
  constraint coincident L0.start A0.centre
  constraint perpendicular L1 L6
  constraint coincident L3.start L6
  constraint perpendicular L3 L6
  constraint perpendicular L3 L4
  constraint perpendicular L5 L6
  constraint collinear L6 L7
  measures "d138" diameter of A0
  measures "d147" distance of L2.start L2.end
  measures "d148" distance of L3.start L3.end
  measures "d149" distance of L3.end L4.end
  measures "d150" distance of L1 L3
  measures "d151" distance of L2 L5
  measures "d152" distance of L3.end L4.end
  measures "d153" distance of L4.end L5.end
  measures "d154" distance of L1.start L1.end
extrude "Extrude1'" add sketch "Sketch9" against normal blind 20 from surface at 66 sketch seen with x (1, 0, 0) y (0, 1, 0) z (0, 0, 1) at (0, -5, 0) bodies 3 in component "Axis"
fillet "Fillet1" radius 5 8 edges at (37.9126, 41, 67.0371) (32.9629, 41, 62.0874) (32.9629, 41, 37.9126) (37.9126, 41, 32.9629) (62.0874, 41, 32.9629) (67.0371, 41, 37.9126) (62.0874, 41, 67.0371) (67.0371, 41, 62.0874) on bodies 3 in component "Axis"
component "Axis" placed x (1, 0, 0) y (0, 1, 0) z (0, 0, 1) at (0, 5, 0)
component "Wheel" placed x (1, 0, 0) y (0, 1, 0) z (0, 0, 1) at (0, 5, 0.5)
equation "d25 = ( 77 / 2 ) * 1 mm"
equation "d33 = ( 77 / 2 ) * 1 mm"

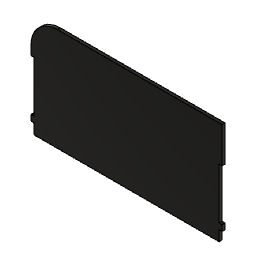
design "Hour Flap"
Autodesk Fusion 360 part; units mm, degrees
sketch "Sketch1" plane through (0, 0, 0) normal (0, 1, 0) x (1, 0, 0)
  line L0 (1, 0) -> (64, 0)
  line L1 (65, -3.5) -> (65, -5.5)
  line L2 (65, -35) -> (9, -35)
  line L3 (1, 0) -> (1, -3.5)
  line L4 (1, -3.5) -> (0, -3.5)
  line L5 (0, -3.5) -> (0, -5.5)
  line L6 (0, -5.5) -> (1, -5.5)
  line L7 (1, -5.5) -> (1, -22.85)
  line L8 (1, -22.85) -> (0, -22.85)
  line L9 (0, -22.85) -> (0, -26)
  arc A0 (0, -26) -> (9, -35) centre (9, -26) ccw
  line L10 (64, -3.5) -> (65, -3.5)
  line L11 (64, -5.5) -> (65, -5.5)
  line L12 (64, -3.5) -> (64, 0)
  line L13 (64, -5.5) -> (64, -22.85)
  line L14 (64, -22.85) -> (65, -22.85)
  line L15 (65, -22.85) -> (65, -35)
  dimension "d3" = 3.5
  dimension "d4" = 2
  dimension "d5" = 17.35
  dimension "d7" = 1
  dimension "d8" = 1
  dimension "d9" = 1
  dimension "d10" = 17.35
  constraint horizontal L0
  constraint vertical L1
  constraint horizontal L2
  constraint vertical L3
  constraint horizontal L4
  constraint perpendicular L4 L5
  constraint perpendicular L6 L7
  constraint perpendicular L7 L8
  constraint perpendicular L2 L9
  constraint perpendicular L1 L10
  constraint perpendicular L1 L11
  constraint perpendicular L11 L13
  constraint perpendicular L13 L14
  measures "d3" distance of origin L4.end
  measures "d4" distance of L4.end L5.end
  measures "d5" distance of L6.end L7.end
  measures "d7" distance of L7.end L8.end
  measures "d8" distance of L5.end L6.end
  measures "d9" distance of L3.end L4.end
  measures "d10" distance of L11.start L13.end
extrude "Extrude1" add sketch "Sketch1" along normal blind 1 makes body 1
copy_body "Body->Comp1" bodies 1 removing the originals makes body 2 in component "Flap"
component "Flap" placed x (1, 0, 0) y (0, 1, 0) z (0, 0, 1) at (0, 0, 0)

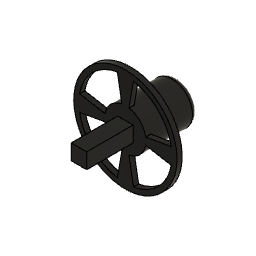
design "Module Connector"
Autodesk Fusion 360 part; units mm, degrees
sketch "Sketch1" plane through (0, 0, 0) normal (0, 1, 0) x (1, 0, 0)
  circle A0 centre (0, 0) radius 4
  dimension "d1" = 8
  constraint coincident A0.centre origin
  measures "d1" diameter of A0
extrude "Extrude1" add sketch "Sketch1" along normal blind 9 makes body 1
sketch "Sketch2" plane through (0, 0, 0) normal (0, 1, 0) x (1, 0, 0)
  line L0 (-0.6946, -3.9392) -> (-1.5628, -8.8633)
  line L1 (0.6946, 3.9392) -> (1.5628, 8.8633)
  line L2 (0.6946, -3.9392) -> (1.5628, -8.8633)
  line L3 (-0.6946, 3.9392) -> (-1.5628, 8.8633)
  line L4 (-3.9392, -0.6946) -> (-8.8633, -1.5628)
  line L5 (-3.9392, 0.6946) -> (-8.8633, 1.5628)
  line L6 (3.9392, -0.6946) -> (8.8633, -1.5628)
  line L7 (3.9392, 0.6946) -> (8.8633, 1.5628)
  arc A0 (-8.8633, -1.5628) -> (-1.5628, -8.8633) centre (0, 0) ccw
  arc A1 (1.5628, -8.8633) -> (8.8633, -1.5628) centre (0, 0) ccw
  arc A2 (8.8633, 1.5628) -> (1.5628, 8.8633) centre (0, 0) ccw
  arc A3 (-1.5628, 8.8633) -> (-8.8633, 1.5628) centre (0, 0) ccw
  arc A4 (3.9392, 0.6946) -> (0.6946, 3.9392) centre (0, 0) ccw
  arc A5 (-0.6946, 3.9392) -> (-3.9392, 0.6946) centre (0, 0) ccw
  arc A6 (-3.9392, -0.6946) -> (-0.6946, -3.9392) centre (0, 0) ccw
  arc A7 (0.6946, -3.9392) -> (3.9392, -0.6946) centre (0, 0) ccw
  dimension "d21" = 18
  constraint perpendicular L3 L7
  constraint coincident L4.end A2
  constraint coincident L0.end A2
  constraint coincident L2.end A2
  constraint concentric A0 A2
  constraint coincident L3.end A2
  constraint concentric A0 A1
  constraint concentric A2 A3
  constraint concentric A4 A6
  constraint concentric A4 A5
  constraint concentric A6 A7
  measures "d21" diameter of A2
fillet "Fillet1" radius 1 1 edges at (-3.7293, 9, 1.4465) on bodies 1
sketch "Sketch3" plane through (0, 0, 0) normal (0, 1, 0) x (1, 0, 0)
  circle A0 centre (0, 0) radius 10
  dimension "d22" = 20
  constraint coincident A0.centre origin
  measures "d22" diameter of A0
extrude "Extrude3" add sketch "Sketch3" against normal blind 1 bodies 1
extrude "Extrude4" cut sketch "Sketch2" against normal blind 1 bodies 1
sketch "Sketch4" plane through (0, -1, 0) normal (0, -1, 0) x (1, 0, 0)
  line L0 (1.5628, -8.8633) -> (0.6946, -3.9392)
  arc A0 (0.6946, -3.9392) -> (3.9392, -0.6946) centre (0, 0) ccw
  line L1 (3.9392, -0.6946) -> (8.8633, -1.5628)
  arc A1 (1.5628, -8.8633) -> (8.8633, -1.5628) centre (0, 0) ccw
  line L2 (-8.8633, -1.5628) -> (-3.9392, -0.6946)
  arc A2 (-3.9392, -0.6946) -> (-0.6946, -3.9392) centre (0, 0) ccw
  line L3 (-0.6946, -3.9392) -> (-1.5628, -8.8633)
  arc A3 (-8.8633, -1.5628) -> (-1.5628, -8.8633) centre (0, 0) ccw
  line L4 (8.8633, 1.5628) -> (3.9392, 0.6946)
  arc A4 (3.9392, 0.6946) -> (0.6946, 3.9392) centre (0, 0) ccw
  line L5 (0.6946, 3.9392) -> (1.5628, 8.8633)
  arc A5 (8.8633, 1.5628) -> (1.5628, 8.8633) centre (0, 0) ccw
  line L6 (-1.5628, 8.8633) -> (-0.6946, 3.9392)
  arc A6 (-0.6946, 3.9392) -> (-3.9392, 0.6946) centre (0, 0) ccw
  line L7 (-3.9392, 0.6946) -> (-8.8633, 1.5628)
  arc A7 (-1.5628, 8.8633) -> (-8.8633, 1.5628) centre (0, 0) ccw
  circle A8 centre (0, 0) radius 10
  line L8 (-1.5, 1.5) -> (1.5, 1.5)
  line L9 (1.5, 1.5) -> (1.5, -1.5)
  line L10 (1.5, -1.5) -> (-1.5, -1.5)
  line L11 (-1.5, -1.5) -> (-1.5, 1.5)
  dimension "d27" = 3
  dimension "d28" = 3
  dimension "d29" = 1.5
  dimension "d30" = 1.5
  constraint horizontal L8
  constraint vertical L9
  constraint horizontal L10
  constraint vertical L11
  measures "d27" distance of L8.start L8.end
  measures "d28" distance of L8.start L10.end
  measures "d29" distance of A0.centre L11
  measures "d30" distance of A0.centre L8
extrude "Extrude5" add sketch "Sketch4" along normal blind 9 contours L8 L9 L10 L11 bodies 1
copy_body "Body->Comp1" bodies 1 removing the originals makes body 2 in component "Component"
component "Component" placed x (1, 0, 0) y (0, 1, 0) z (0, 0, 1) at (0, 0, 0)

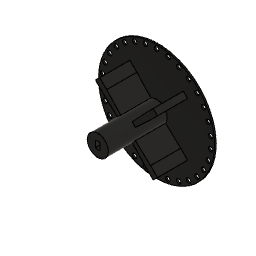
design "Minute Wheel 2"
Autodesk Fusion 360 part; units mm, degrees
sketch "Sketch1" plane through (0, 0, 0) normal (0, 1, 0) x (1, 0, 0)
  circle A0 centre (0, 0) radius 38.5
  circle A1 centre (0, -36) radius 1.5
  circle A2 centre (7.4848, -35.2133) radius 1.5
  circle A3 centre (14.6425, -32.8876) radius 1.5
  circle A4 centre (21.1603, -29.1246) radius 1.5
  circle A5 centre (26.7532, -24.0887) radius 1.5
  circle A6 centre (31.1769, -18) radius 1.5
  circle A7 centre (34.238, -11.1246) radius 1.5
  circle A8 centre (35.8028, -3.763) radius 1.5
  circle A9 centre (35.8028, 3.763) radius 1.5
  circle A10 centre (34.238, 11.1246) radius 1.5
  circle A11 centre (31.1769, 18) radius 1.5
  circle A12 centre (26.7532, 24.0887) radius 1.5
  circle A13 centre (21.1603, 29.1246) radius 1.5
  circle A14 centre (14.6425, 32.8876) radius 1.5
  circle A15 centre (7.4848, 35.2133) radius 1.5
  circle A16 centre (0, 36) radius 1.5
  circle A17 centre (-7.4848, 35.2133) radius 1.5
  circle A18 centre (-14.6425, 32.8876) radius 1.5
  circle A19 centre (-21.1603, 29.1246) radius 1.5
  circle A20 centre (-26.7532, 24.0887) radius 1.5
  circle A21 centre (-31.1769, 18) radius 1.5
  circle A22 centre (-34.238, 11.1246) radius 1.5
  circle A23 centre (-35.8028, 3.763) radius 1.5
  circle A24 centre (-35.8028, -3.763) radius 1.5
  circle A25 centre (-34.238, -11.1246) radius 1.5
  circle A26 centre (-31.1769, -18) radius 1.5
  circle A27 centre (-26.7532, -24.0887) radius 1.5
  circle A28 centre (-21.1603, -29.1246) radius 1.5
  circle A29 centre (-14.6425, -32.8876) radius 1.5
  circle A30 centre (-7.4848, -35.2133) radius 1.5
  dimension "d1" = 77
  dimension "d94" = 3
  dimension "d95" = 36
  dimension "d97" = 360
  constraint coincident A0.centre origin
  measures "d1" diameter of A0
  measures "d94" diameter of A1
  measures "d95" distance of A0.centre A1.centre
extrude "Extrude1" add sketch "Sketch1" along normal blind 1 makes body 1
sketch "Sketch2" plane through (0, 0, 0) normal (0, 1, 0) x (1, 0, 0)
  line L0 (0, 0) -> (27.6586, 0) construction
  line L1 (0, 0) -> (41.0195, 0) construction
  line L2 (0, 0) -> (31, 0) construction
  line L3 (0, 0) -> (31, 0) construction
  line L4 (-15.9765, 13.148) -> (-13.148, 15.9765)
  line L5 (-14.5622, 14.5622) -> (-15.9765, 13.148)
  line L6 (-14.5622, 14.5622) -> (-13.148, 15.9765)
  line L7 (-15.9765, 13.148) -> (-20.5726, 17.7442)
  line L8 (-20.5726, 17.7442) -> (-17.7442, 20.5726)
  line L9 (-13.148, 15.9765) -> (-17.7442, 20.5726)
  line L10 (-15.9765, -13.148) -> (-20.5726, -17.7442)
  line L11 (-14.5622, -14.5622) -> (-13.148, -15.9765)
  line L12 (-13.148, -15.9765) -> (-17.7442, -20.5726)
  line L13 (-17.7442, -20.5726) -> (-20.5726, -17.7442)
  line L14 (-14.5622, -14.5622) -> (-15.9765, -13.148)
  line L15 (-13.148, -15.9765) -> (-15.9765, -13.148)
  line L16 (13.148, -15.9765) -> (17.7442, -20.5726)
  line L17 (14.5622, -14.5622) -> (15.9765, -13.148)
  line L18 (15.9765, -13.148) -> (20.5726, -17.7442)
  line L19 (20.5726, -17.7442) -> (17.7442, -20.5726)
  line L20 (14.5622, -14.5622) -> (13.148, -15.9765)
  line L21 (15.9765, -13.148) -> (13.148, -15.9765)
  line L22 (15.9765, 13.148) -> (20.5726, 17.7442)
  line L23 (14.5622, 14.5622) -> (13.148, 15.9765)
  line L24 (13.148, 15.9765) -> (17.7442, 20.5726)
  line L25 (17.7442, 20.5726) -> (20.5726, 17.7442)
  line L26 (14.5622, 14.5622) -> (15.9765, 13.148)
  line L27 (13.148, 15.9765) -> (15.9765, 13.148)
  line L28 (-15.9765, 13.148) -> (-5.9061, 3.7573)
  line L29 (-15.9765, 13.148) -> (0.824, 13.148) construction
  line L30 (-13.148, 15.9765) -> (-3.7573, 5.9061)
  line L31 (-13.148, 15.9765) -> (3.6363, 15.9765) construction
  line L32 (13.148, 15.9765) -> (3.7573, 5.9061)
  line L33 (13.148, 15.9765) -> (30.0166, 15.9765) construction
  line L34 (15.9765, 13.148) -> (5.9061, 3.7573)
  line L35 (15.9765, 13.148) -> (32.7225, 13.148) construction
  line L36 (-15.9765, -13.148) -> (-5.9061, -3.7573)
  line L37 (-15.9765, -13.148) -> (0.8229, -13.148) construction
  line L38 (-13.148, -15.9765) -> (-3.7573, -5.9061)
  line L39 (-13.148, -15.9765) -> (3.6463, -15.9765) construction
  line L40 (15.9765, -13.148) -> (5.9061, -3.7573)
  line L41 (15.9765, -13.148) -> (32.8382, -13.148) construction
  line L42 (13.148, -15.9765) -> (3.7573, -5.9061)
  line L43 (13.148, -15.9765) -> (30.0097, -15.9765) construction
  line L44 (-3.6455, 1.6463) -> (-3.6903, 1.691)
  line L45 (-3.6901, -1.6909) -> (-3.6455, -1.6463)
  line L46 (1.9993, -0.0019) -> (1.9974, 0)
  line L47 (-1.6458, 3.6457) -> (-1.7011, 3.7012)
  line L48 (3.6463, 1.6445) -> (3.7292, 1.7273)
  line L49 (-1.6943, -3.6938) -> (-1.6461, -3.6456)
  line L50 (1.9993, -0.0019) -> (2.0012, 0)
  arc A0 (3.7573, -5.9061) -> (5.9061, -3.7573) centre (0, 0) ccw
  arc A1 (5.9061, 3.7573) -> (3.7573, 5.9061) centre (0, 0) ccw
  arc A2 (-3.7573, 5.9061) -> (-5.9061, 3.7573) centre (0, 0) ccw
  arc A3 (-5.9061, -3.7573) -> (-3.7573, -5.9061) centre (0, 0) ccw
  dimension "d26" = 2
  dimension "d27" = 2
  dimension "d28" = 6.5
  dimension "d29" = 4
  dimension "d30" = 27.0941
  dimension "d32" = 360
  dimension "d64" = 43
  dimension "d65" = 47
  dimension "d66" = 133
  dimension "d67" = 137
  dimension "d68" = 43
  dimension "d69" = 47
  dimension "d70" = 137
  dimension "d71" = 133
  dimension "d91" = 14
  constraint horizontal L0
  constraint coincident L0.start L1.start
  constraint horizontal L1
  constraint horizontal L2
  constraint horizontal L3
  constraint perpendicular L4 L7
  constraint perpendicular L8 L9
  constraint coincident L4 L5.start
  constraint horizontal L29
  constraint horizontal L31
  constraint horizontal L33
  constraint horizontal L35
  constraint horizontal L37
  constraint horizontal L39
  constraint horizontal L41
  constraint horizontal L43
  constraint coincident L47.start L46
  constraint coincident L48.start L49
  constraint collinear L46 L47
  constraint coincident L0 L50.end
  constraint collinear L48 L49
  constraint coincident L0 L46.end
  constraint coincident L46.start L49
  constraint collinear L49 L50
  constraint coincident L36.end A0
  constraint concentric A0 A1
  constraint concentric A1 A2
  constraint concentric A2 A3
  measures "d26" distance of L5.start L4.start
  measures "d27" distance of L5.start L4.end
  measures "d28" distance of L4.start L7.end
  measures "d29" distance of L7.end L8.end
  measures "d30" distance of L0.start L8
  measures "d64" angle of L28 L29
  measures "d65" angle of L30 L31
  measures "d66" angle of L32 L33
  measures "d67" angle of L34 L35
  measures "d68" angle of L36 L37
  measures "d69" angle of L38 L39
  measures "d70" angle of L40 L41
  measures "d71" angle of L42 L43
  measures "d91" diameter of A0
extrude "Extrude2" add sketch "Sketch2" against normal blind 20 bodies 1